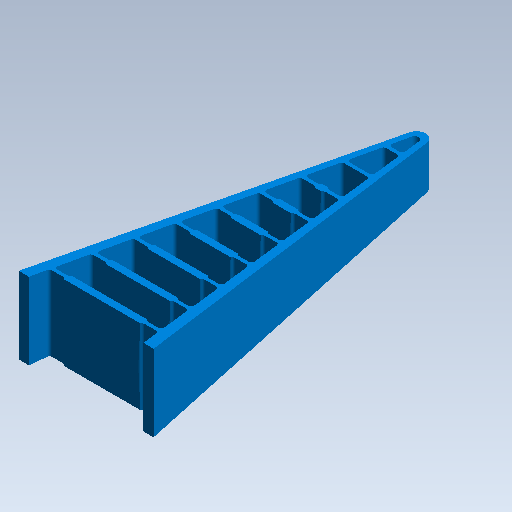
# Autodesk Inventor part: 3998964 DHAS-GF-80-U-BU
Saved by Autodesk Inventor 2020 (Build 240168000, 168)
## iProperties
Part Number: 3998964 DHAS-GF-80-U-BU
Material: Generic
Catalog Web Link: www.cadenas.de
Description: DHAS-GF-Adaptive Gripper Finger
Vendor: FESTO
Document SubType Name: Modeling
Designer: partserver
Manufacturer: FESTO
Mass: 13 g
Surface Area: 129.078 cm^2
Volume: 11.9169 cm^3
Density: 1 g/cm^3
Appearance: PSOLRGB-0-153-255
Category: PARTsolutions
Company: FESTO
PSOL_IDENT_0: {$CADENAS_DATA\23d-libs\festo\parts\d\dhas\dhas_gf.prj},188 {VTYP=3D},{NB=3998964 DHAS-GF-80-U-BU},{
PSOL_IDENT_1: LINA=3998964 DHAS-GF-80-U-BU},{NN=DHAS-GF},{DATE=27.04.2020 13:53:14},{GEOMDATE=30.08.2019 14:47:40}
PSOL_IDENT_2: ,{VERSION=},{LINEID=230},{WBVAR=},{WBNUMERIC=}  {NB=3998964 DHAS-GF-80-U-BU},{LINA=3998964 DHAS-GF-8
PSOL_IDENT_3: 0-U-BU},{KT=DUMMY},{TNR=3998964},{TYP=DHAS-GF-80-U-BU},{L=94.5},{CNSMASSEXACT=0.0130},{B1=21.337}
NB: 3998964 DHAS-GF-80-U-BU
NN: DHAS-GF
NT: Adaptive Gripper Finger
NBSYN: $TNR. $TYP.
LINA: 3998964 DHAS-GF-80-U-BU
CATALOG: Festo
TNR: 3998964
TYP: DHAS-GF-80-U-BU
L: 94.5
CNSMASSEXACT: 0.013
SUPPLIER: FESTO
ARTICLENO: 3998964 DHAS-GF-80-U-BU
BOMINFO: 3998964 DHAS-GF-80-U-BU
CREATOR: CADENAS GmbH
Title: 3998964 DHAS-GF-80-U-BU
Author: Cadenas PARTsolutions
Comments: Adaptive Gripper Finger
Autodesk Inventor part; units mm, degrees
ref_plane "YZ Plane" through (0, 0, 0) normal (1, 0, 0) x (0, 1, 0)
ref_plane "XZ Plane" through (0, 0, 0) normal (0, 1, 0) x (-1, 0, 0)
ref_plane "XY Plane" through (0, 0, 0) normal (0, 0, 1) x (1, 0, 0)
sketch "Sketch_1" plane through (0, 0, 0) normal (0, 0, 1) x (1, 0, 0)
  line L0 (-18.761, 0) -> (-15.92, 0)
  line L1 (-15.92, 0) -> (-15.217986, 4.328086)
  arc A0 (-14.428306, 5) -> (-15.217986, 4.328086) centre (-14.428306, 4.2) ccw
  line L2 (-14.428306, 5) -> (-11.360371, 5)
  arc A1 (-10.795, 4.766) -> (-11.360371, 5) centre (-11.360371, 4.2) ccw
  line L3 (-10.795, 4.766) -> (-10.582, 4.552)
  arc A2 (-10.582, 4.552) -> (-10.016629, 4.318) centre (-10.016629, 5.118) ccw
  line L4 (-10.016629, 4.318) -> (10.016629, 4.318)
  arc A3 (10.016629, 4.318) -> (10.582, 4.552) centre (10.016629, 5.118) ccw
  line L5 (10.582, 4.552) -> (10.795, 4.766)
  arc A4 (11.360371, 5) -> (10.795, 4.766) centre (11.360371, 4.2) ccw
  line L6 (11.360371, 5) -> (14.428306, 5)
  arc A5 (15.217986, 4.328086) -> (14.428306, 5) centre (14.428306, 4.2) ccw
  line L7 (15.217986, 4.328086) -> (15.92, 0)
  line L8 (15.92, 0) -> (18.761, 0)
  line L9 (18.761, 0) -> (2.461978, 92.434124)
  arc A6 (2.461978, 92.434124) -> (-2.461978, 92.434124) centre (0, 91.99977) ccw
  line L10 (-2.461978, 92.434124) -> (-18.761, 0)
  arc A7 (-1.833, 86.927999) -> (-1.043306, 86) centre (-1.043306, 86.8) ccw
  line L11 (-1.043306, 86) -> (1.043306, 86)
  arc A8 (1.043306, 86) -> (1.833, 86.927999) centre (1.043306, 86.8) ccw
  line L12 (1.833, 86.927999) -> (1.066, 91.66)
  arc A9 (1.066, 91.66) -> (0, 92.567) centre (0.008483, 91.497034) ccw
  arc A10 (0, 92.567) -> (-1.066, 91.66) centre (-0.008483, 91.497034) ccw
  line L13 (-1.066, 91.66) -> (-1.833, 86.927999)
  arc A11 (-3.454008, 76.927953) -> (-2.664306, 76) centre (-2.664306, 76.8) ccw
  line L14 (-2.664306, 76) -> (2.664306, 76)
  arc A12 (2.664306, 76) -> (3.454008, 76.927953) centre (2.664306, 76.8) ccw
  line L15 (3.454008, 76.927953) -> (2.255008, 84.327953)
  arc A13 (2.255008, 84.327953) -> (1.465306, 85) centre (1.465306, 84.2) ccw
  line L16 (1.465306, 85) -> (-1.465306, 85)
  arc A14 (-1.465306, 85) -> (-2.255008, 84.327953) centre (-1.465306, 84.2) ccw
  line L17 (-2.255008, 84.327953) -> (-3.454008, 76.927953)
  arc A15 (-5.074008, 66.927953) -> (-4.284306, 66) centre (-4.284306, 66.8) ccw
  line L18 (-4.284306, 66) -> (-1.691371, 66)
  arc A16 (-1.691371, 66) -> (-1.125686, 66.234314) centre (-1.691371, 66.8) ccw
  line L19 (-1.125686, 66.234314) -> (-0.713314, 66.646686)
  arc A17 (-0.147629, 66.881) -> (-0.713314, 66.646686) centre (-0.147629, 66.081) ccw
  line L20 (-0.147629, 66.881) -> (0.147629, 66.881)
  arc A18 (0.713314, 66.646686) -> (0.147629, 66.881) centre (0.147629, 66.081) ccw
  line L21 (0.713314, 66.646686) -> (1.125686, 66.234314)
  arc A19 (1.125686, 66.234314) -> (1.691371, 66) centre (1.691371, 66.8) ccw
  line L22 (1.691371, 66) -> (4.284306, 66)
  arc A20 (4.284306, 66) -> (5.074008, 66.927953) centre (4.284306, 66.8) ccw
  line L23 (5.074008, 66.927953) -> (3.875008, 74.327953)
  arc A21 (3.875008, 74.327953) -> (3.085306, 75) centre (3.085306, 74.2) ccw
  line L24 (3.085306, 75) -> (-3.085306, 75)
  arc A22 (-3.085306, 75) -> (-3.875008, 74.327953) centre (-3.085306, 74.2) ccw
  line L25 (-3.875008, 74.327953) -> (-5.074008, 66.927953)
  arc A23 (-6.695008, 56.927953) -> (-5.905306, 56) centre (-5.905306, 56.8) ccw
  line L26 (-5.905306, 56) -> (-3.302371, 56)
  arc A24 (-3.302371, 56) -> (-2.736045, 56.234958) centre (-3.302372, 56.8) ccw
  line L27 (-2.736045, 56.234958) -> (-2.29725, 56.67525)
  arc A25 (-1.731629, 56.91) -> (-2.29725, 56.67525) centre (-1.731129, 56.11) ccw
  line L28 (-1.731629, 56.91) -> (1.731629, 56.91)
  arc A26 (2.29725, 56.67525) -> (1.731629, 56.91) centre (1.731129, 56.11) ccw
  line L29 (2.29725, 56.67525) -> (2.737, 56.234)
  arc A27 (2.737, 56.234) -> (3.302371, 56) centre (3.302371, 56.8) ccw
  line L30 (3.302371, 56) -> (5.905306, 56)
  arc A28 (5.905306, 56) -> (6.695008, 56.927953) centre (5.905306, 56.8) ccw
  line L31 (6.695008, 56.927953) -> (5.496008, 64.327953)
  arc A29 (5.496008, 64.327953) -> (4.706306, 65) centre (4.706306, 64.2) ccw
  line L32 (4.706306, 65) -> (1.691371, 65)
  arc A30 (1.691371, 65) -> (1.126, 64.766) centre (1.691371, 64.2) ccw
  line L33 (1.126, 64.766) -> (0.966, 64.605)
  arc A31 (0.400629, 64.371) -> (0.966, 64.605) centre (0.400629, 65.171) ccw
  line L34 (0.400629, 64.371) -> (-0.400629, 64.371)
  arc A32 (-0.966, 64.605) -> (-0.400629, 64.371) centre (-0.400629, 65.171) ccw
  line L35 (-0.966, 64.605) -> (-1.126, 64.766)
  arc A33 (-1.126, 64.766) -> (-1.691371, 65) centre (-1.691371, 64.2) ccw
  line L36 (-1.691371, 65) -> (-4.706306, 65)
  arc A34 (-4.706306, 65) -> (-5.496008, 64.327953) centre (-4.706306, 64.2) ccw
  line L37 (-5.496008, 64.327953) -> (-6.695008, 56.927953)
  arc A35 (-8.315008, 46.927953) -> (-7.525306, 46) centre (-7.525306, 46.8) ccw
  line L38 (-7.525306, 46) -> (-4.914371, 46)
  arc A36 (-4.914371, 46) -> (-4.348686, 46.234314) centre (-4.914371, 46.8) ccw
  line L39 (-4.348686, 46.234314) -> (-3.881315, 46.701685)
  arc A37 (-3.31563, 46.936) -> (-3.881315, 46.701685) centre (-3.315629, 46.136) ccw
  line L40 (-3.31563, 46.936) -> (3.31563, 46.936)
  arc A38 (3.881315, 46.701685) -> (3.31563, 46.936) centre (3.315629, 46.136) ccw
  line L41 (3.881315, 46.701685) -> (4.348686, 46.234314)
  arc A39 (4.348686, 46.234314) -> (4.914371, 46) centre (4.914371, 46.8) ccw
  line L42 (4.914371, 46) -> (7.525306, 46)
  arc A40 (7.525306, 46) -> (8.315008, 46.927953) centre (7.525306, 46.8) ccw
  line L43 (8.315008, 46.927953) -> (7.116008, 54.327953)
  arc A41 (7.116008, 54.327953) -> (6.326306, 55) centre (6.326306, 54.2) ccw
  line L44 (6.326306, 55) -> (3.302371, 55)
  arc A42 (3.302371, 55) -> (2.737, 54.766) centre (3.302371, 54.2) ccw
  line L45 (2.737, 54.766) -> (2.569001, 54.595002)
  arc A43 (2.002629, 54.36) -> (2.569001, 54.595002) centre (2.002629, 55.16) ccw
  line L46 (2.002629, 54.36) -> (-2.002629, 54.36)
  arc A44 (-2.569001, 54.595002) -> (-2.002629, 54.36) centre (-2.002629, 55.16) ccw
  line L47 (-2.569001, 54.595002) -> (-2.737, 54.766)
  arc A45 (-2.737, 54.766) -> (-3.302371, 55) centre (-3.302371, 54.2) ccw
  line L48 (-3.302371, 55) -> (-6.326306, 55)
  arc A46 (-6.326306, 55) -> (-7.116008, 54.327953) centre (-6.326306, 54.2) ccw
  line L49 (-7.116008, 54.327953) -> (-8.315008, 46.927953)
  arc A47 (-9.936008, 36.927953) -> (-9.146306, 36) centre (-9.146306, 36.8) ccw
  line L50 (-9.146306, 36) -> (-6.526371, 36)
  arc A48 (-6.526371, 36) -> (-5.961, 36.234) centre (-6.526371, 36.8) ccw
  line L51 (-5.961, 36.234) -> (-5.471862, 36.7311)
  arc A49 (-4.901629, 36.97) -> (-5.471862, 36.7311) centre (-4.901628, 36.17) ccw
  line L52 (-4.901629, 36.97) -> (4.901629, 36.97)
  arc A50 (5.471862, 36.7311) -> (4.901629, 36.97) centre (4.901628, 36.17) ccw
  line L53 (5.471862, 36.7311) -> (5.961, 36.234)
  arc A51 (5.961, 36.234) -> (6.526371, 36) centre (6.526371, 36.8) ccw
  line L54 (6.526371, 36) -> (9.146306, 36)
  arc A52 (9.146306, 36) -> (9.936008, 36.927953) centre (9.146306, 36.8) ccw
  line L55 (9.936008, 36.927953) -> (8.737008, 44.327953)
  arc A53 (8.737008, 44.327953) -> (7.947306, 45) centre (7.947306, 44.2) ccw
  line L56 (7.947306, 45) -> (4.914371, 45)
  arc A54 (4.914371, 45) -> (4.348686, 44.765686) centre (4.914371, 44.2) ccw
  line L57 (4.348686, 44.765686) -> (4.170315, 44.587315)
  arc A55 (3.60463, 44.353) -> (4.170315, 44.587315) centre (3.604629, 45.153) ccw
  line L58 (3.60463, 44.353) -> (-3.60463, 44.353)
  arc A56 (-4.170315, 44.587315) -> (-3.60463, 44.353) centre (-3.604629, 45.153) ccw
  line L59 (-4.170315, 44.587315) -> (-4.348686, 44.765686)
  arc A57 (-4.348686, 44.765686) -> (-4.914371, 45) centre (-4.914371, 44.2) ccw
  line L60 (-4.914371, 45) -> (-7.947306, 45)
  arc A58 (-7.947306, 45) -> (-8.737008, 44.327953) centre (-7.947306, 44.2) ccw
  line L61 (-8.737008, 44.327953) -> (-9.936008, 36.927953)
  arc A59 (-11.556008, 26.927953) -> (-10.766306, 26) centre (-10.766306, 26.8) ccw
  line L62 (-10.766306, 26) -> (-8.137371, 26)
  arc A60 (-8.137371, 26) -> (-7.571686, 26.234314) centre (-8.137371, 26.8) ccw
  line L63 (-7.571686, 26.234314) -> (-7.051315, 26.754685)
  arc A61 (-6.48563, 26.989) -> (-7.051315, 26.754685) centre (-6.485629, 26.189) ccw
  line L64 (-6.48563, 26.989) -> (6.48563, 26.989)
  arc A62 (7.051315, 26.754685) -> (6.48563, 26.989) centre (6.485629, 26.189) ccw
  line L65 (7.051315, 26.754685) -> (7.571686, 26.234314)
  arc A63 (7.571686, 26.234314) -> (8.137371, 26) centre (8.137371, 26.8) ccw
  line L66 (8.137371, 26) -> (10.766306, 26)
  arc A64 (10.766306, 26) -> (11.556008, 26.927953) centre (10.766306, 26.8) ccw
  line L67 (11.556008, 26.927953) -> (10.357008, 34.327953)
  arc A65 (10.357008, 34.327953) -> (9.567306, 35) centre (9.567306, 34.2) ccw
  line L68 (9.567306, 35) -> (6.526371, 35)
  arc A66 (6.526371, 35) -> (5.960685, 34.765685) centre (6.526371, 34.2) ccw
  line L69 (5.960685, 34.765685) -> (5.773315, 34.578315)
  arc A67 (5.20763, 34.344) -> (5.773315, 34.578315) centre (5.207629, 35.144) ccw
  line L70 (5.20763, 34.344) -> (-5.20763, 34.344)
  arc A68 (-5.773315, 34.578315) -> (-5.20763, 34.344) centre (-5.207629, 35.144) ccw
  line L71 (-5.773315, 34.578315) -> (-5.960685, 34.765685)
  arc A69 (-5.960685, 34.765685) -> (-6.526371, 35) centre (-6.526371, 34.2) ccw
  line L72 (-6.526371, 35) -> (-9.567306, 35)
  arc A70 (-9.567306, 35) -> (-10.357008, 34.327953) centre (-9.567306, 34.2) ccw
  line L73 (-10.357008, 34.327953) -> (-11.556008, 26.927953)
  arc A71 (-13.176991, 16.928057) -> (-12.387306, 16) centre (-12.387306, 16.8) ccw
  line L74 (-12.387306, 16) -> (-9.749371, 16)
  arc A72 (-9.749371, 16) -> (-9.183685, 16.234315) centre (-9.749371, 16.8) ccw
  line L75 (-9.183685, 16.234315) -> (-8.637314, 16.780686)
  arc A73 (-8.071629, 17.015) -> (-8.637314, 16.780686) centre (-8.071629, 16.215) ccw
  line L76 (-8.071629, 17.015) -> (8.071629, 17.015)
  arc A74 (8.637314, 16.780686) -> (8.071629, 17.015) centre (8.071629, 16.215) ccw
  line L77 (8.637314, 16.780686) -> (9.183685, 16.234315)
  arc A75 (9.183685, 16.234315) -> (9.749371, 16) centre (9.749371, 16.8) ccw
  line L78 (9.749371, 16) -> (12.387306, 16)
  arc A76 (12.387306, 16) -> (13.176991, 16.928057) centre (12.387306, 16.8) ccw
  line L79 (13.176991, 16.928057) -> (11.976991, 24.328057)
  arc A77 (11.976991, 24.328057) -> (11.187306, 25) centre (11.187306, 24.2) ccw
  line L80 (11.187306, 25) -> (8.137371, 25)
  arc A78 (8.137371, 25) -> (7.571686, 24.765686) centre (8.137371, 24.2) ccw
  line L81 (7.571686, 24.765686) -> (7.375315, 24.569315)
  arc A79 (6.80963, 24.335) -> (7.375315, 24.569315) centre (6.809629, 25.135) ccw
  line L82 (6.80963, 24.335) -> (-6.80963, 24.335)
  arc A80 (-7.375315, 24.569315) -> (-6.80963, 24.335) centre (-6.809629, 25.135) ccw
  line L83 (-7.375315, 24.569315) -> (-7.571686, 24.765686)
  arc A81 (-7.571686, 24.765686) -> (-8.137371, 25) centre (-8.137371, 24.2) ccw
  line L84 (-8.137371, 25) -> (-11.187306, 25)
  arc A82 (-11.187306, 25) -> (-11.976991, 24.328057) centre (-11.187306, 24.2) ccw
  line L85 (-11.976991, 24.328057) -> (-13.176991, 16.928057)
  arc A83 (-14.797008, 6.927953) -> (-14.007306, 6) centre (-14.007306, 6.8) ccw
  line L86 (-14.007306, 6) -> (-11.360371, 6)
  arc A84 (-11.360371, 6) -> (-10.794193, 6.234808) centre (-11.360372, 6.8) ccw
  line L87 (-10.794193, 6.234808) -> (-10.222807, 6.807192)
  arc A85 (-9.656629, 7.042) -> (-10.222807, 6.807192) centre (-9.656628, 6.242) ccw
  line L88 (-9.656629, 7.042) -> (9.656629, 7.042)
  arc A86 (10.222807, 6.807192) -> (9.656629, 7.042) centre (9.656628, 6.242) ccw
  line L89 (10.222807, 6.807192) -> (10.794193, 6.234808)
  arc A87 (10.794193, 6.234808) -> (11.360371, 6) centre (11.360372, 6.8) ccw
  line L90 (11.360371, 6) -> (14.007306, 6)
  arc A88 (14.007306, 6) -> (14.797008, 6.927953) centre (14.007306, 6.8) ccw
  line L91 (14.797008, 6.927953) -> (13.598008, 14.327953)
  arc A89 (13.598008, 14.327953) -> (12.808306, 15) centre (12.808306, 14.2) ccw
  line L92 (12.808306, 15) -> (9.749371, 15)
  arc A90 (9.749371, 15) -> (9.183685, 14.765685) centre (9.749371, 14.2) ccw
  line L93 (9.183685, 14.765685) -> (8.979314, 14.561314)
  arc A91 (8.413629, 14.327) -> (8.979314, 14.561314) centre (8.413629, 15.127) ccw
  line L94 (8.413629, 14.327) -> (-8.413629, 14.327)
  arc A92 (-8.979314, 14.561314) -> (-8.413629, 14.327) centre (-8.413629, 15.127) ccw
  line L95 (-8.979314, 14.561314) -> (-9.183685, 14.765685)
  arc A93 (-9.183685, 14.765685) -> (-9.749371, 15) centre (-9.749371, 14.2) ccw
  line L96 (-9.749371, 15) -> (-12.808306, 15)
  arc A94 (-12.808306, 15) -> (-13.598008, 14.327953) centre (-12.808306, 14.2) ccw
  line L97 (-13.598008, 14.327953) -> (-14.797008, 6.927953)
  constraints: 196 end point, 190 point on circle, 95 centre point
extrude "Extrusion1" add sketch "Sketch_1" along normal mid plane 31.337
sketch "Sketch_2" plane through (0, 0, 0) normal (1, 0, 0) x (0, 1, 0)
  line L0 (104.5, 21.337) -> (-10, 21.337)
  line L1 (-10, 21.337) -> (-10, -21.337)
  line L2 (-10, -21.337) -> (104.5, -21.337)
  line L3 (104.5, -21.337) -> (104.5, 21.337)
  line L4 (0, 10.6685) -> (0, -10.6685)
  line L5 (0, -10.6685) -> (94.5, -5.881337)
  line L6 (94.5, -5.881337) -> (94.5, 5.881337)
  line L7 (94.5, 5.881337) -> (0, 10.6685)
  constraints: 16 end point
extrude "Extrusion2" cut sketch "Sketch_2" along normal mid plane 70
sketch "Sketch_3" plane through (0, 0, 0) normal (1, 0, 0) x (0, 1, 0)
  line L0 (9, 20) -> (4, 20)
  line L1 (4, 20) -> (4, -20)
  line L2 (4, -20) -> (9, -20)
  line L3 (9, -20) -> (9, 20)
  line L4 (4.5, 10.44054) -> (4.31776, 0)
  line L5 (4.31776, 0) -> (4.5, -10.44054)
  line L6 (4.5, -10.44054) -> (6.5, -10.339224)
  line L7 (6.5, -10.339224) -> (7.041856, 0)
  line L8 (7.041856, 0) -> (6.5, 10.339224)
  line L9 (6.5, 10.339224) -> (4.5, 10.44054)
  constraints: 20 end point
extrude "Extrusion3" cut sketch "Sketch_3" along normal mid plane 24
sketch "Sketch_4" plane through (0, 0, 0) normal (1, 0, 0) x (0, 1, 0)
  line L0 (18, 20) -> (13, 20)
  line L1 (13, 20) -> (13, -20)
  line L2 (13, -20) -> (18, -20)
  line L3 (18, -20) -> (18, 20)
  line L4 (14.5, 9.933962) -> (14.326602, 0)
  line L5 (14.326602, 0) -> (14.5, -9.933962)
  line L6 (14.5, -9.933962) -> (16.5, -9.832646)
  line L7 (16.5, -9.832646) -> (17.015307, 0)
  line L8 (17.015307, 0) -> (16.5, 9.832646)
  line L9 (16.5, 9.832646) -> (14.5, 9.933962)
  constraints: 20 end point
extrude "Extrusion4" cut sketch "Sketch_4" along normal mid plane 20
sketch "Sketch_5" plane through (0, 0, 0) normal (1, 0, 0) x (0, 1, 0)
  line L0 (28, 20) -> (23, 20)
  line L1 (23, 20) -> (23, -20)
  line L2 (23, -20) -> (28, -20)
  line L3 (28, -20) -> (28, 20)
  line L4 (24.5, 9.427384) -> (24.335444, 0)
  line L5 (24.335444, 0) -> (24.5, -9.427384)
  line L6 (24.5, -9.427384) -> (26.5, -9.326068)
  line L7 (26.5, -9.326068) -> (26.988759, 0)
  line L8 (26.988759, 0) -> (26.5, 9.326068)
  line L9 (26.5, 9.326068) -> (24.5, 9.427384)
  constraints: 20 end point
extrude "Extrusion5" cut sketch "Sketch_5" along normal mid plane 18
sketch "Sketch_6" plane through (0, 0, 0) normal (1, 0, 0) x (0, 1, 0)
  line L0 (38, 20) -> (33, 20)
  line L1 (33, 20) -> (33, -20)
  line L2 (33, -20) -> (38, -20)
  line L3 (38, -20) -> (38, 20)
  line L4 (34.5, 8.920805) -> (34.344287, 0)
  line L5 (34.344287, 0) -> (34.5, -8.920805)
  line L6 (34.5, -8.920805) -> (36.5, -8.81949)
  line L7 (36.5, -8.81949) -> (36.96221, 0)
  line L8 (36.96221, 0) -> (36.5, 8.81949)
  line L9 (36.5, 8.81949) -> (34.5, 8.920805)
  constraints: 20 end point
extrude "Extrusion6" cut sketch "Sketch_6" along normal mid plane 16
sketch "Sketch_7" plane through (0, 0, 0) normal (1, 0, 0) x (0, 1, 0)
  line L0 (48, 20) -> (43, 20)
  line L1 (43, 20) -> (43, -20)
  line L2 (43, -20) -> (48, -20)
  line L3 (48, -20) -> (48, 20)
  line L4 (44.5, 8.414227) -> (44.353129, 0)
  line L5 (44.353129, 0) -> (44.5, -8.414227)
  line L6 (44.5, -8.414227) -> (46.5, -8.312912)
  line L7 (46.5, -8.312912) -> (46.935661, 0)
  line L8 (46.935661, 0) -> (46.5, 8.312912)
  line L9 (46.5, 8.312912) -> (44.5, 8.414227)
  constraints: 20 end point
extrude "Extrusion7" cut sketch "Sketch_7" along normal mid plane 14
sketch "Sketch_8" plane through (0, 0, 0) normal (1, 0, 0) x (0, 1, 0)
  line L0 (58, 20) -> (53, 20)
  line L1 (53, 20) -> (53, -20)
  line L2 (53, -20) -> (58, -20)
  line L3 (58, -20) -> (58, 20)
  line L4 (54.5, 7.907649) -> (54.361971, 0)
  line L5 (54.361971, 0) -> (54.5, -7.907649)
  line L6 (54.5, -7.907649) -> (56.5, -7.806333)
  line L7 (56.5, -7.806333) -> (56.909113, 0)
  line L8 (56.909113, 0) -> (56.5, 7.806333)
  line L9 (56.5, 7.806333) -> (54.5, 7.907649)
  constraints: 20 end point
extrude "Extrusion8" cut sketch "Sketch_8" along normal mid plane 8
sketch "Sketch_9" plane through (0, 0, 0) normal (1, 0, 0) x (0, 1, 0)
  line L0 (68, 20) -> (63, 20)
  line L1 (63, 20) -> (63, -20)
  line L2 (63, -20) -> (68, -20)
  line L3 (68, -20) -> (68, 20)
  line L4 (64.5, 7.401071) -> (64.370814, 0)
  line L5 (64.370814, 0) -> (64.5, -7.401071)
  line L6 (64.5, -7.401071) -> (66.5, -7.299755)
  line L7 (66.5, -7.299755) -> (66.882564, 0)
  line L8 (66.882564, 0) -> (66.5, 7.299755)
  line L9 (66.5, 7.299755) -> (64.5, 7.401071)
  constraints: 20 end point
extrude "Extrusion9" cut sketch "Sketch_9" along normal mid plane 4
body "Solid1"
